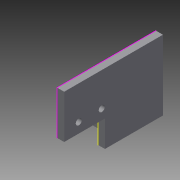
# Autodesk Inventor part: bart y end stop bracket plain switch v1
Saved by Autodesk Inventor 2014 SP1 (Build 180222100, 222)
## iProperties
Created: 2015-06-04
Part Number: bart y end stop bracket plain switch v1
Material: Generic
Document SubType Name: Modeling
Designer: Mon
Density: 1 g/cm^3
Appearance: Default
Author: Mon
Autodesk Inventor part; units mm, degrees
sketch "Sketch1" plane through (0, 0, 0) normal (0, 0, 1) x (1, 0, 0)
  line L0 (0, 0) -> (16.5, 0)
  line L1 (16.5, 0) -> (16.5, -24)
  line L2 (16.5, -24) -> (0, -24)
  line L3 (0, -24) -> (0, 0)
  line L4 (24.2611, -12.002) -> (-7.0214, -12.002)
  circle A0 centre (4.1138, -12.002) radius 2
  dimension "d0" = 16.5
  dimension "d1" = 24
  dimension "d7" = 4
  constraints: 10 end point, 2 parallel, 2 perpendicular, 1 centre point, 1 horizontal, 1 point on line
  measures "d0" distance of L1.end L2.end
  measures "d1" distance of L0.end L1.end
  measures "d7" diameter of A0
ref_plane "Work Plane2" through (16.5, -24, 0) normal (1, 0, 0) x (0, 0, -1)
sketch "Sketch2" plane through (16.5, -24, 0) normal (1, 0, 0) x (0, 0, -1)
  line L0 (-3, -16.8669) -> (-3, 24)
  line L1 (-3, -16.8669) -> (-23, -16.8669)
  line L2 (-23, -16.8669) -> (5.9335, -16.8669)
  line L3 (5.9335, -16.8669) -> (5.9335, 24)
  line L4 (5.9335, 24) -> (-23, 24)
  line L5 (-23, 24) -> (-23, -16.8669)
  circle A0 centre (-9.1835, -1.3253) radius 1.25
  line L6 (-9.1835, -1.3253) -> (-9.1835, -10.8253) construction
  circle A1 centre (-9.1835, -10.8253) radius 1.25
  dimension "d11" = 20
  dimension "d12" = 2.5
  dimension "d13" = 9.5
  dimension "d14" = 2.5
  constraints: 14 end point, 4 parallel, 2 centre point, 2 perpendicular, 1 coincident, 1 horizontal
  measures "d11" distance of L0.start L1.end
  measures "d12" diameter of A0
  measures "d13" distance of L6.start L6.end
  measures "d14" diameter of A1
extrude "Extrusion2" add sketch "Sketch2" along normal blind 3
ref_plane "Work Plane3" through (16.5, -24, 0) normal (-1, 0, 0) x (0, 0, 1)
sketch "Sketch3" plane through (16.5, -24, 0) normal (-1, 0, 0) x (0, 0, 1)
  line L0 (-5.9335, -16.8669) -> (-5.9335, 24) projected
  line L1 (-5.9335, 0.0047) -> (4.9967, 0.0047)
  line L2 (4.9967, 0.0047) -> (4.9967, -16.8669)
  line L3 (4.9967, -16.8669) -> (-5.9335, -16.8669)
  line L4 (-5.9335, -16.8669) -> (-5.9335, 0.0047)
  constraints: 8 end point, 2 parallel, 1 horizontal, 1 perpendicular, 1 point on line
extrude "Extrusion3" cut sketch "Sketch3" against normal through all
ref_plane "Work Plane1" through (0, -7, 3) normal (0, 1, 0) x (1, 0, 0)
sketch "Sketch4" plane through (16.5, -24, 0) normal (-1, 0, 0) x (0, 0, 1)
  line L0 (4.9967, 0.0047) -> (4.9967, -16.8669) projected
  line L1 (23, -16.8669) -> (4.9967, -16.8669) projected
  line L2 (23, 24) -> (23, -16.8669) projected
  line L3 (3, 24) -> (23, 24) projected
  line L4 (3, 0.0047) -> (3, 24) projected
  line L5 (3, 0.0047) -> (4.9967, 0.0047) projected
  line L6 (4.9967, 0.0047) -> (4.9967, -16.8669) projected
  line L7 (23, -16.8669) -> (4.9967, -16.8669) projected
  line L8 (23, 24) -> (23, -16.8669) projected
  line L9 (-5.9335, 24) -> (23, 24) projected
  line L10 (-5.9335, 0.0047) -> (-5.9335, 24) projected
  line L11 (-5.9335, 0.0047) -> (4.9967, 0.0047) projected
  point P0 (0, 24)
extrude "Extrusion4" add sketch "Sketch1" along normal blind 3 contours L0 L1 L4 A0 L3 | L4 A0 L1 L2 L3
sketch "Sketch5" plane through (0, -7, 3) normal (0, 1, 0) x (1, 0, 0)
  line L0 (3.8833, -0.0391) -> (16.3772, -10.1018)
  line L1 (16.3772, -10.1018) -> (16.3772, -0.0391)
  line L2 (16.3772, -0.0391) -> (3.8833, -0.0391)
  point P0 (0, 3)
  constraints: 6 end point, 1 perpendicular, 1 vertical
extrude "Extrusion5" add sketch "Sketch5" along normal blind 3
body "Solid1"
